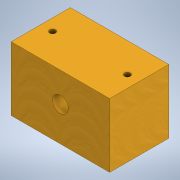
# Autodesk Inventor part: Pin Block
Saved by Autodesk Inventor 2020.4 (Build 244396000, 396)
## iProperties
Created: 2022-04-16
Part Number: Pin Block
Material: Brass, Soft Yellow, Welded
Document SubType Name: Modeling
Designer: Gurkin
Density: 8.5 g/cm^3
Appearance: Weld - Brass
Author: Gurkin
Autodesk Inventor part; units mm, degrees
ref_plane "YZ Plane" through (0, 0, 0) normal (1, 0, 0) x (0, 1, 0)
ref_plane "XZ Plane" through (0, 0, 0) normal (0, 1, 0) x (-1, 0, 0)
ref_plane "XY Plane" through (0, 0, 0) normal (0, 0, 1) x (1, 0, 0)
sketch "Sketch1" plane through (0, 0, 0) normal (0, 0, 1) x (1, 0, 0)
  line L0 (-36, 33) -> (64, 33)
  line L1 (64, 33) -> (64, -32)
  line L2 (64, -32) -> (-36, -32)
  line L3 (-36, -32) -> (-36, 33)
  point P0 (0, 0)
  dimension "d0" = 100
  dimension "d1" = 65
  constraints: 8 end point, 2 parallel, 1 horizontal, 1 perpendicular
  measures "d0" distance between parallel lines of L1 L3
  measures "d1" distance between parallel lines of L2 L0
extrude "Extrusion1" add sketch "Sketch1" along normal blind 60
sketch "Sketch2" plane through (0, 0, 60) normal (0, 0, 1) x (1, 0, 0)
  circle A0 centre (14, 3) radius 8
  line L0 (64, 33) -> (-36, 33) projected
  line L1 (64, -32) -> (64, 33) projected
  line L2 (-36, -32) -> (64, -32) projected
  point P0 (0, 0)
  dimension "d4" = 16
  dimension "d6" = 50
  dimension "d7" = 35
  constraints: 1 centre point
  measures "d4" diameter of A0
  measures "d6" distance from line of L1 A0.centre
  measures "d7" distance from line of L2 A0.centre
extrude "Extrusion2" cut sketch "Sketch2" against normal through all
sketch "Sketch3" plane through (-36, 33, 0) normal (0, 1, 0) x (1, 0, 0)
  circle A0 centre (12, -30) radius 3
  line L0 (100, 0) -> (0, 0) projected
  line L1 (0, 0) -> (0, -60) projected
  circle A1 centre (88, -30) radius 3
  line L2 (100, 0) -> (100, -60) projected
  point P0 (36, 0)
  dimension "d10" = 6
  dimension "d11" = 30
  dimension "d12" = 12
  dimension "d13" = 6
  dimension "d14" = 30
  dimension "d15" = 12
  constraints: 2 centre point
  measures "d10" diameter of A0
  measures "d11" distance from line of L0 A0.centre
  measures "d12" distance from line of L1 A0.centre
  measures "d13" diameter of A1
  measures "d14" distance from line of L0 A1.centre
  measures "d15" distance from line of L2 A1.centre
extrude "Extrusion3" cut sketch "Sketch3" against normal through all
body "Solid1"
